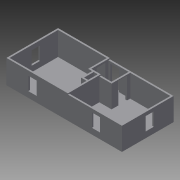
# Autodesk Inventor part: 489 Forest 2nd Floor
Saved by Autodesk Inventor 2013 SP2 (Build 170200200, 200)
## iProperties
Created: 2014-06-02
Part Number: 489 Forest 2nd Floor
Material: Generic
Document SubType Name: Modeling
Designer: jmw3
Density: 1 g/cm^3
Author: jmw3
Autodesk Inventor part; units mm, degrees
ref_plane "YZ Plane" through (0, 0, 0) normal (1, 0, 0) x (0, 1, 0)
ref_plane "XZ Plane" through (0, 0, 0) normal (0, 1, 0) x (-1, 0, 0)
ref_plane "XY Plane" through (0, 0, 0) normal (0, 0, 1) x (1, 0, 0)
sketch "Sketch1" plane through (0, 0, 0) normal (0, 1, 0) x (-1, 0, 0)
  line L0 (2008.4767, 2311.4) -> (5359.4, 2311.4)
  line L1 (-5511.8, 2463.8) -> (1195.6767, 2463.8)
  line L2 (2008.4767, 2463.8) -> (5511.8, 2463.8)
  line L3 (5359.4, 2311.4) -> (5359.4, -2311.4)
  line L4 (128.8767, 2311.4) -> (1195.6767, 2311.4)
  line L5 (2008.4767, 2311.4) -> (5359.4, 2311.4)
  line L6 (-5359.4, 2311.4) -> (-1041.4, 2311.4)
  line L7 (-5359.4, -2311.4) -> (-5359.4, 2311.4)
  line L8 (-988.7233, -2463.8) -> (-5306.7233, -2463.8)
  line L9 (5359.4, -2311.4) -> (1955.8, -2311.4)
  line L10 (355.6, -2463.8) -> (1143, -2463.8)
  line L11 (1955.8, -2463.8) -> (5359.4, -2463.8)
  line L12 (5359.4, 2311.4) -> (5359.4, -2311.4)
  line L13 (-5359.4, -2311.4) -> (-5359.4, 2311.4)
  line L14 (128.8767, 2311.4) -> (1195.6767, 2311.4)
  line L15 (-5359.4, 2311.4) -> (-1041.4, 2311.4)
  line L16 (1955.8, -2311.4) -> (5359.4, -2311.4)
  line L17 (5359.4, -2311.4) -> (5359.4, 2311.4)
  line L18 (5359.4, 2311.4) -> (2008.4767, 2311.4)
  line L19 (2008.4767, 2463.8) -> (5511.8, 2463.8)
  line L20 (-457.2, -2463.8) -> (-457.2, -2311.4)
  line L21 (355.6, -2463.8) -> (355.6, -2311.4)
  line L22 (-7716.52, 0) -> (7716.52, 0) projected
  line L23 (-5511.8, 2463.8) -> (-5511.8, -2463.8)
  line L24 (-5306.7233, -2463.8) -> (-5511.8, -2463.8)
  line L25 (5511.8, 2463.8) -> (5511.8, -2463.8)
  line L26 (5511.8, -2463.8) -> (5359.4, -2463.8)
  line L27 (-988.7233, -2463.8) -> (-457.2, -2463.8)
  line L28 (-1371.6, -685.8) -> (558.8, -685.8)
  line L29 (558.8, -2311.4) -> (355.6, -2311.4)
  line L30 (-457.2, -2311.4) -> (-1371.6, -2311.4)
  line L31 (-1371.6, -2311.4) -> (-457.2, -2311.4)
  line L32 (355.6, -2311.4) -> (558.8, -2311.4)
  line L33 (-355.6, -533.4) -> (-355.6, 2311.4)
  line L34 (1143, -2311.4) -> (1955.8, -2311.4)
  line L35 (1955.8, -2463.8) -> (1143, -2463.8)
  line L36 (0, -3449.32) -> (0, 3449.32) projected
  line L37 (1195.6767, 2463.8) -> (2008.4767, 2463.8)
  line L38 (2008.4767, 2311.4) -> (1195.6767, 2311.4)
  line L39 (355.6, -2463.8) -> (5511.8, -2463.8)
  line L40 (1143, -2311.4) -> (711.2, -2311.4)
  line L41 (558.8, -2311.4) -> (355.6, -2311.4)
  line L42 (-1041.4, -2311.4) -> (-1371.6, -2311.4)
  line L43 (-1524, -2311.4) -> (-5359.4, -2311.4)
  line L44 (-203.2, 533.4) -> (330.2, 533.4)
  line L45 (330.2, 533.4) -> (330.2, -533.4)
  line L46 (-1524, -2006.6) -> (-1371.6, -2006.6)
  line L47 (-1524, -1193.8) -> (-1371.6, -1193.8)
  line L48 (558.8, -1193.8) -> (711.2, -1193.8)
  line L49 (558.8, -2006.6) -> (711.2, -2006.6)
  line L50 (-1371.6, -2311.4) -> (-1371.6, -2006.6)
  line L51 (-1371.6, -1193.8) -> (-1371.6, -685.8)
  line L52 (-1524, -533.4) -> (-1524, -1193.8)
  line L53 (-1524, -2006.6) -> (-1524, -2311.4)
  line L54 (558.8, -685.8) -> (558.8, -1193.8)
  line L55 (558.8, -2006.6) -> (558.8, -2311.4)
  line L56 (711.2, -2311.4) -> (711.2, -2006.6)
  line L57 (711.2, -1193.8) -> (711.2, -533.4)
  line L58 (-203.2, -533.4) -> (177.8, -533.4)
  line L59 (177.8, -533.4) -> (177.8, 381)
  line L60 (177.8, 381) -> (-203.2, 381)
  line L61 (-203.2, 381) -> (-203.2, -533.4)
  line L62 (1195.6767, 2311.4) -> (-203.2, 2311.4)
  line L63 (-355.6, 2311.4) -> (-5359.4, 2311.4)
  line L64 (-23.5233, 2311.4) -> (-203.2, 2311.4)
  line L65 (-355.6, 2311.4) -> (-889, 2311.4)
  line L66 (-889, 2311.4) -> (-355.6, 2311.4)
  line L67 (-203.2, 2311.4) -> (-23.5233, 2311.4)
  line L68 (-203.2, 2311.4) -> (-203.2, 533.4)
  line L69 (-203.2, 381) -> (-203.2, -533.4)
  line L70 (711.2, -533.4) -> (330.2, -533.4)
  line L71 (177.8, -533.4) -> (-203.2, -533.4)
  line L72 (-355.6, -533.4) -> (-1524, -533.4)
  point P0 (0, 0)
  point P1 (0, 0)
  dimension "d0" = 152.4
  dimension "d8" = 152.4
  dimension "d12" = 11023.6
  dimension "d14" = 152.4
  dimension "d15" = 152.4
  dimension "d23" = 5054.6
  dimension "d29" = 4927.6
  dimension "d30" = 152.4
  dimension "d32" = 5029.2
  dimension "d33" = 304.8
  dimension "d34" = 1117.6
  dimension "d35" = 304.8
  dimension "d36" = 1117.6
  dimension "d37" = 152.4
  dimension "d38" = 3835.4
  dimension "d40" = 152.4
  dimension "d41" = 812.8
  dimension "d42" = 4648.2
  dimension "d73" = 152.4
  dimension "d74" = 152.4
  dimension "d75" = 152.4
  dimension "d77" = 2844.8
  dimension "d78" = 152.4
  dimension "d79" = 5562.6
  dimension "d80" = 1778
  constraints: 142 end point, 33 parallel, 26 collinear, 25 perpendicular, 9 horizontal, 2 other
  measures "d0" distance between parallel lines of L2 L0
  measures "d8" distance between parallel lines of L9 L11
  measures "d12" distance between parallel lines of L25 L23
  measures "d14" distance between parallel lines of L25 L17
  measures "d15" distance between parallel lines of L23 L7
  measures "d23" distance between parallel lines of L23 L20
  measures "d29" distance between parallel lines of L11 L2
  measures "d30" distance between parallel lines of L43 L8
  measures "d32" distance between parallel lines of L3 L45
  measures "d33" distance between parallel lines of L43 L46
  measures "d34" distance between parallel lines of L43 L47
  measures "d35" distance from line of L34.start L49
  measures "d36" distance between parallel lines of L34 L48
  measures "d37" distance between parallel lines of L51 L52
  measures "d38" distance between parallel lines of L7 L52
  measures "d40" distance between parallel lines of L57 L54
  measures "d41" distance between parallel lines of L20 L21
  measures "d42" distance between parallel lines of L3 L57
  measures "d73" distance between parallel lines of L44 L60
  measures "d74" distance between parallel lines of L45 L59
  measures "d75" distance between parallel lines of L33 L68
  measures "d77" distance between parallel lines of L6 L72
  measures "d78" distance between parallel lines of L28 L72
  measures "d79" distance between parallel lines of L3 L68
  measures "d80" distance between parallel lines of L62 L44
extrude "Extrusion12" add sketch "Sketch1" along normal blind 2133.6 contours L38 L4 L62 L36 L1 L37 L2 L25 L22 L3 L0 | L22 L25 L26 L11 L35 L10 L21 L29 L55 L49 L56 L40 L34 L9 L3 | L45 L70 L57 L48 L54 L28 L36 L58 L59 L22 | L22 L59 L60 L36 L44 L45 | L62 L68 L44 L36 L60 L61 L22 L33 L63 L6 L7 L23 L1 | L61 L58 L36 L28 L51 L47 L52 L72 L33 L22 | L22 L7 L43 L53 L46 L50 L30 L20 L27 L8 L24 L23
sketch "Sketch10" plane through (0, 0, 0) normal (0, -1, 0) x (1, 0, 0)
  line L0 (-5511.8, 2463.8) -> (5511.8, 2463.8)
  line L1 (5511.8, 2463.8) -> (5511.8, -2463.8)
  line L2 (5511.8, -2463.8) -> (-5511.8, -2463.8)
  line L3 (-5511.8, -2463.8) -> (-5511.8, 2463.8)
  point P0 (0, 0)
  constraints: 8 end point, 2 parallel, 1 horizontal, 1 perpendicular
extrude "Extrusion13" add sketch "Sketch10" along normal blind 25.4
sketch "Sketch11" plane through (0, 2133.6, 0) normal (0, 1, 0) x (1, 0, 0)
  line L0 (1371.6, 685.8) -> (-558.8, 685.8) projected
  line L1 (-355.6, 2463.8) -> (-5511.8, 2463.8) projected
  line L2 (355.6, 533.4) -> (355.6, 685.8)
  line L3 (-558.8, 2463.8) -> (-558.8, 2311.4)
  line L4 (-558.8, 2006.6) -> (-711.2, 2006.6)
  line L5 (-711.2, 2006.6) -> (-711.2, 1193.8)
  line L6 (-711.2, 1193.8) -> (-558.8, 1193.8)
  line L7 (-558.8, 1193.8) -> (-558.8, 2006.6)
  line L8 (1371.6, 1193.8) -> (1524, 1193.8)
  line L9 (1524, 1193.8) -> (1524, 2006.6)
  line L10 (1524, 2006.6) -> (1371.6, 2006.6)
  line L11 (1371.6, 2006.6) -> (1371.6, 1193.8)
  line L12 (-5511.8, -2463.8) -> (5511.8, -2463.8) projected
  line L13 (355.6, -2311.4) -> (355.6, -2463.8)
  line L14 (203.2, 533.4) -> (203.2, -381) projected
  line L15 (203.2, -381) -> (-177.8, -381) projected
  line L16 (-177.8, -381) -> (-177.8, 533.4) projected
  line L17 (-177.8, 533.4) -> (203.2, 533.4) projected
  line L18 (-5511.8, -2463.8) -> (5511.8, -2463.8) projected
  line L19 (5511.8, -2463.8) -> (5511.8, 2463.8) projected
  line L20 (5511.8, 2463.8) -> (457.2, 2463.8) projected
  line L21 (457.2, 2463.8) -> (457.2, 2311.4) projected
  line L22 (457.2, 2311.4) -> (1371.6, 2311.4) projected
  line L23 (1371.6, 2311.4) -> (1371.6, 2006.6) projected
  line L24 (1371.6, 2006.6) -> (1524, 2006.6) projected
  line L25 (1524, 2006.6) -> (1524, 2311.4) projected
  line L26 (1524, 2311.4) -> (5359.4, 2311.4) projected
  line L27 (5359.4, 2311.4) -> (5359.4, -2311.4) projected
  line L28 (5359.4, -2311.4) -> (355.6, -2311.4) projected
  line L29 (355.6, -2311.4) -> (355.6, 533.4) projected
  line L30 (355.6, 533.4) -> (1524, 533.4) projected
  line L31 (1524, 533.4) -> (1524, 1193.8) projected
  line L32 (1524, 1193.8) -> (1371.6, 1193.8) projected
  line L33 (1371.6, 1193.8) -> (1371.6, 685.8) projected
  line L34 (1371.6, 685.8) -> (-558.8, 685.8) projected
  line L35 (-558.8, 685.8) -> (-558.8, 1193.8) projected
  line L36 (-558.8, 1193.8) -> (-711.2, 1193.8) projected
  line L37 (-711.2, 1193.8) -> (-711.2, 533.4) projected
  line L38 (-711.2, 533.4) -> (-330.2, 533.4) projected
  line L39 (-330.2, 533.4) -> (-330.2, -533.4) projected
  line L40 (-330.2, -533.4) -> (203.2, -533.4) projected
  line L41 (203.2, -533.4) -> (203.2, -2311.4) projected
  line L42 (203.2, -2311.4) -> (-5359.4, -2311.4) projected
  line L43 (-5359.4, -2311.4) -> (-5359.4, 2311.4) projected
  line L44 (-5359.4, 2311.4) -> (-711.2, 2311.4) projected
  line L45 (-711.2, 2311.4) -> (-711.2, 2006.6) projected
  line L46 (-711.2, 2006.6) -> (-558.8, 2006.6) projected
  line L47 (-558.8, 2006.6) -> (-558.8, 2311.4) projected
  line L48 (-355.6, 2311.4) -> (-355.6, 2463.8) projected
  line L49 (-355.6, 2463.8) -> (-5511.8, 2463.8) projected
  line L50 (-5511.8, 2463.8) -> (-5511.8, -2463.8) projected
  line L51 (-558.8, 2006.6) -> (-558.8, 2463.8)
  line L52 (355.6, 685.8) -> (355.6, -2463.8)
  line L53 (355.6, 685.8) -> (-558.8, 685.8)
  line L54 (-558.8, 685.8) -> (-558.8, 2463.8)
  line L55 (-330.2, 533.4) -> (-330.2, -533.4) projected
  line L56 (-558.8, 2463.8) -> (-711.2, 2463.8)
  line L57 (-711.2, 2463.8) -> (-711.2, 533.4)
  line L58 (-711.2, 533.4) -> (-558.8, 533.4)
  line L59 (-558.8, 533.4) -> (-558.8, 2463.8)
  line L60 (-558.8, 533.4) -> (355.6, 533.4)
  line L61 (355.6, 533.4) -> (355.6, 685.8)
  line L62 (355.6, 685.8) -> (-558.8, 685.8)
  line L63 (-558.8, 685.8) -> (-558.8, 533.4)
  line L64 (355.6, 685.8) -> (203.2, 685.8)
  line L65 (203.2, 685.8) -> (203.2, -2463.8)
  line L66 (203.2, -2463.8) -> (355.6, -2463.8)
  line L67 (355.6, -2463.8) -> (355.6, 685.8)
  line L68 (203.2, -533.4) -> (-330.2, -533.4)
  line L69 (-330.2, -533.4) -> (-330.2, -368.3)
  line L70 (-330.2, -368.3) -> (203.2, -368.3)
  line L71 (203.2, -368.3) -> (203.2, -533.4)
  line L72 (-330.2, 533.4) -> (-177.8, 533.4)
  line L73 (-177.8, 533.4) -> (-177.8, -533.4)
  line L74 (-177.8, -533.4) -> (-330.2, -533.4)
  line L75 (-330.2, -533.4) -> (-330.2, 533.4)
  line L76 (-558.8, 2311.4) -> (-5511.8, 2311.4)
  line L77 (-5511.8, 2311.4) -> (-5511.8, 2463.8)
  line L78 (-5511.8, 2463.8) -> (-558.8, 2463.8)
  line L79 (-558.8, 2463.8) -> (-558.8, 2311.4)
  line L80 (-558.8, 2311.4) -> (-355.6, 2311.4) projected
  line L81 (-355.6, 2463.8) -> (457.2, 2463.8)
  line L82 (457.2, 2463.8) -> (457.2, 2311.4)
  line L83 (457.2, 2311.4) -> (-355.6, 2311.4)
  line L84 (-355.6, 2311.4) -> (-355.6, 2463.8)
  point P0 (0, 2298.7)
  point P1 (0, 2451.1)
  point P2 (0, 0)
  constraints: 86 end point, 19 parallel, 12 perpendicular, 9 horizontal, 5 point on line, 3 collinear, 2 other
extrude "Extrusion15" add sketch "Sketch11" against normal blind 76.2 contours L11 L10 L9 L8 | L6 L5 L4 L7
extrude "Extrusion16" add sketch "Sketch11" along normal blind 101.6 contours L2 L60 L65 L0 | L65 L17 L60 L38 L59 L0 | L29 L13 L12 L65 L41 L14 L60 | L59 L38 L37 L6 L35 | L6 L5 L4 L7 | L16 L70 L39 L60 | L4 L45 L76 L47 | L65 L40 L73 L15 | L16 L73 L40 L39 L70 | L12 L50 L76 L43 L42 L65 | L76 L57 L1 L3 | L44 L76 L50 L1 L57
extrude "Extrusion17" add sketch "Sketch11" along normal blind 101.6 contours L2 L60 L65 L0 | L65 L17 L60 L38 L59 L0
sketch "Sketch12" plane through (5511.8, 2133.6, 2463.8) normal (1, 0, 0) x (0, 0, -1)
  line L0 (4927.6, -2159) -> (4927.6, 0) projected
  line L1 (0, 0) -> (4927.6, 0) projected
  line L2 (4775.2, -2133.6) -> (152.4, -2133.6) projected
  line L3 (4775.2, -2133.6) -> (152.4, -2133.6) projected
  line L4 (152.4, -2133.6) -> (152.4, 0) projected
  line L5 (4775.2, 0) -> (152.4, 0) projected
  line L6 (4775.2, -2133.6) -> (4775.2, 0) projected
  line L7 (2260.6, -330.2) -> (3048, -330.2)
  line L8 (3048, -330.2) -> (3048, -1600.2)
  line L9 (3048, -1600.2) -> (2260.6, -1600.2)
  line L10 (2260.6, -1600.2) -> (2260.6, -330.2)
  point P0 (2463.8, -2133.6)
  dimension "d93" = 1879.6
  dimension "d94" = 787.4
  dimension "d95" = 330.2
  dimension "d96" = 533.4
  constraints: 8 end point, 2 parallel, 1 horizontal, 1 perpendicular
  measures "d93" distance between parallel lines of L0 L8
  measures "d94" distance between parallel lines of L8 L10
  measures "d95" distance between parallel lines of L1 L7
  measures "d96" distance between parallel lines of L2 L9
extrude "Extrusion18" cut sketch "Sketch12" against normal up to surface (152.4 mm away) contours L7 L8 L9 L10
sketch "Sketch13" plane through (5359.4, 2133.6, 2311.4) normal (0, 0, -1) x (-1, 0, 0)
  line L0 (0, -2133.6) -> (5003.8, -2133.6) projected
  line L1 (0, 0) -> (5003.8, 0) projected
  line L2 (-152.4, -2159) -> (-152.4, 0) projected
  line L3 (5003.8, 0) -> (-152.4, 0) projected
  line L4 (5003.8, 0) -> (5003.8, 101.6) projected
  line L5 (10871.2, 101.6) -> (5003.8, 101.6) projected
  line L6 (10871.2, 101.6) -> (10871.2, -2159) projected
  line L7 (-152.4, -2159) -> (10871.2, -2159) projected
  line L8 (1930.4, -330.2) -> (2717.8, -330.2)
  line L9 (2717.8, -330.2) -> (2717.8, -1600.2)
  line L10 (2717.8, -1600.2) -> (1930.4, -1600.2)
  line L11 (1930.4, -1600.2) -> (1930.4, -330.2)
  point P0 (5359.4, -2133.6)
  dimension "d99" = 2082.8
  dimension "d100" = 787.4
  dimension "d101" = 330.2
  dimension "d102" = 533.4
  constraints: 8 end point, 2 parallel, 1 horizontal, 1 perpendicular
  measures "d99" distance between parallel lines of L2 L11
  measures "d100" distance between parallel lines of L11 L9
  measures "d101" distance between parallel lines of L1 L8
  measures "d102" distance between parallel lines of L0 L10
extrude "Extrusion19" cut sketch "Sketch13" against normal up to surface (152.4 mm away) contours L8 L9 L10 L11
mirror "Mirror3" about plane through (0, 0, 0) normal (1, 0, 0) of "Extrusion18", "Extrusion19"
extrude "Extrusion20" add sketch "Sketch11" against normal blind 203.2 contours L83 L48 L81 L21
body "Solid2"
